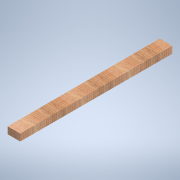
# Autodesk Inventor part: Madera
Saved by Autodesk Inventor 2022 (Build 260153000, 153)
## iProperties
Created: 2022-04-18
Part Number: Madera
Material: Genérico
Document SubType Name: Modeling
Designer: aarco
Density: 1 g/cm^3
Appearance: Valor por defecto
Author: aarco
Autodesk Inventor part; units mm, degrees
ref_plane "YZ Plane" through (0, 0, 0) normal (1, 0, 0) x (0, 1, 0)
ref_plane "XZ Plane" through (0, 0, 0) normal (0, 1, 0) x (-1, 0, 0)
ref_plane "XY Plane" through (0, 0, 0) normal (0, 0, 1) x (1, 0, 0)
sketch "Boceto1" plane through (0, 0, 0) normal (0, 1, 0) x (-1, 0, 0)
  line L0 (34, 411.5) -> (-34, 411.5)
  line L1 (-34, 411.5) -> (-34, -411.5)
  line L2 (-34, -411.5) -> (34, -411.5)
  line L3 (34, -411.5) -> (34, 411.5)
  line L4 (0, 0) -> (0, 553.1756)
  line L5 (0, 0) -> (291.1825, 0)
  dimension "d0" = 823
  dimension "d1" = 68
  constraints: 12 end point, 2 horizontal, 2 parallel, 2 symmetric about line, 1 perpendicular, 1 vertical
  measures "d0" distance of L2.end L0.start
  measures "d1" distance of L0.start L0.end
extrude "Extrusión1" add sketch "Boceto1" along normal blind 37
